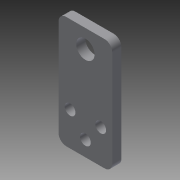
# Autodesk Inventor part: Plaque support
Saved by Autodesk Inventor 2015 SP1 (Build 190203100, 203)
## iProperties
Created: 2015-04-11
Part Number: Plaque support
Material: Generic
Document SubType Name: Modeling
Designer: Cyril
Density: 1 g/cm^3
Appearance: Default
Author: Cyril
Autodesk Inventor part; units mm, degrees
ref_plane "YZ Plane" through (0, 0, 0) normal (1, 0, 0) x (0, 1, 0)
ref_plane "XZ Plane" through (0, 0, 0) normal (0, 1, 0) x (-1, 0, 0)
ref_plane "XY Plane" through (0, 0, 0) normal (0, 0, 1) x (1, 0, 0)
sketch "Sketch1" plane through (0, 0, 0) normal (0, 0, 1) x (1, 0, 0)
  line L0 (-17.5, 36.5) -> (17.5, 36.5)
  line L1 (17.5, 36.5) -> (17.5, -36.5)
  line L2 (17.5, -36.5) -> (-17.5, -36.5)
  line L3 (-17.5, -36.5) -> (-17.5, 36.5)
  line L4 (-17.5, 36.5) -> (17.5, -36.5) construction
  line L5 (17.5, 36.5) -> (-17.5, -36.5) construction
  circle A0 centre (-10, -14.5) radius 3.5
  circle A1 centre (0, -26.5) radius 3.5
  circle A2 centre (10, -14.5) radius 3.5
  circle A3 centre (0, 24.5) radius 6
  line L6 (0, 36.5) -> (0, -36.5) construction
  point P0 (0, 0)
  dimension "d3" = 35
  dimension "d4" = 7
  dimension "d5" = 7
  dimension "d6" = 7
  dimension "d9" = 10
  dimension "d12" = 12
  dimension "d13" = 12
  dimension "d32" = 20
  dimension "d33" = 12
  dimension "d34" = 39
  constraints: 14 end point, 4 centre point, 4 midpoint, 2 parallel, 2 point on line, 1 horizontal, 1 horizontal alignment, 1 perpendicular, 1 symmetric about line
  measures "d3" distance of L0.start L0.end
  measures "d4" diameter of A0
  measures "d5" diameter of A1
  measures "d6" diameter of A2
  measures "d9" distance from line of A1.centre L2
  measures "d12" diameter of A3
  measures "d13" distance from line of L0 A3.centre
  measures "d32" distance of A2.centre A0.centre
  measures "d33" vertical distance of A0.centre A1.centre
  measures "d34" vertical distance of A0.centre A3.centre
extrude "Extrusion3" add sketch "Sketch1" along normal blind 6
fillet "Fillet2" radius 5 4 edges at (-17.5, 36.5, 3) (-17.5, -36.5, 3) (17.5, -36.5, 3) (17.5, 36.5, 3)
equation "\"d5\" = d4"
equation "\"d6\" = d4"
body "Solid3"
